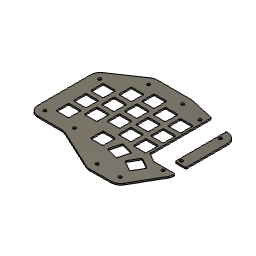
Fifi_Case_v6 (Autodesk Fusion 360 design; units mm, degrees)
Autodesk Fusion 360 part; units mm, degrees
(part 1 of 3)
sketch "top_plate" plane through (0, 0, 0) normal (0, 1, 0) x (1, 0, 0)
  arc A0 (-12.05, -31.06) -> (-13.05, -32.06) centre (-13.05, -31.06) cw
  arc A1 (-45.1, -12) -> (-44.1, -11) centre (-44.1, -12) cw
  arc A2 (-45.1, -4.95) -> (-44.1, -5.95) centre (-44.1, -4.95) ccw
  arc A3 (48.9038, -42.3878) -> (47.5378, -42.7538) centre (48.4038, -43.2538) ccw
  arc A4 (32.1, -35.05) -> (31.1, -34.05) centre (32.1, -34.05) cw
  line L0 (20.8727, -52.5986) -> (32.4638, -55.7044)
  arc A5 (41.5378, -53.1462) -> (41.9038, -54.5122) centre (42.4038, -53.6462) ccw
  line L1 (-25.05, 1) -> (-13.05, 1)
  line L2 (-32.1, 8.05) -> (-44.1, 8.05)
  line L3 (-25.05, 20.05) -> (-13.05, 20.05)
  arc A6 (-25.05, -32.06) -> (-26.05, -31.06) centre (-25.05, -31.06) cw
  arc A7 (36.7944, -43.4062) -> (36.0873, -42.1814) centre (35.8285, -43.1474) ccw
  line L4 (-45.1, -24) -> (-45.1, -12)
  arc A8 (44.1, -2) -> (45.1, -3) centre (44.1, -3) cw
  arc A9 (-12.05, -12) -> (-13.05, -13) centre (-13.05, -12) cw
  arc A10 (31.1, -22.05) -> (32.1, -21.05) centre (32.1, -22.05) cw
  arc A11 (44.1, -21.05) -> (45.1, -22.05) centre (44.1, -22.05) cw
  line L5 (-32.1, -44.05) -> (-44.1, -44.05)
  arc A12 (-32.1, -30.05) -> (-31.1, -31.05) centre (-32.1, -31.05) cw
  line L6 (-44.1, -5.95) -> (-32.1, -5.95)
  line L7 (47.5378, -42.7538) -> (41.5378, -53.1462)
  line L8 (-45.1, 7.05) -> (-45.1, -4.95)
  arc A13 (-45.1, -31.05) -> (-44.1, -30.05) centre (-44.1, -31.05) cw
  line L9 (23.2714, -39.7827) -> (20.1656, -51.3738)
  arc A14 (-25.05, 6.05) -> (-26.05, 7.05) centre (-25.05, 7.05) cw
  arc A15 (-31.1, 7.05) -> (-32.1, 8.05) centre (-32.1, 7.05) ccw
  arc A16 (-31.1, -24) -> (-32.1, -25) centre (-32.1, -24) cw
  arc A17 (32.4638, -55.7044) -> (33.6886, -54.9973) centre (32.7226, -54.7385) ccw
  line L10 (26.1407, -56.1073) -> (17.1311, -53.6931)
  arc A18 (-26.05, 0) -> (-25.05, 1) centre (-25.05, 0) cw
  line L11 (-31.1, -12) -> (-31.1, -24)
  line L12 (44.1, 3.05) -> (32.1, 3.05)
  line L13 (33.6886, -54.9973) -> (36.7944, -43.4062)
  arc A19 (-12.05, 7.05) -> (-13.05, 6.05) centre (-13.05, 7.05) cw
  line L14 (-8.525, 28.075) -> (0, 28.075)
  line L15 (-13.05, 6.05) -> (-25.05, 6.05)
  line L16 (-45.1, -43.05) -> (-45.1, -31.05)
  line L17 (-12.05, 0) -> (-12.05, -12)
  arc A20 (45.1, 4.05) -> (44.1, 3.05) centre (44.1, 4.05) cw
  arc A21 (-13.05, -18.06) -> (-12.05, -19.06) centre (-13.05, -19.06) cw
  line L18 (-12.05, -19.06) -> (-12.05, -31.06)
  arc A22 (-13.05, 1) -> (-12.05, 0) centre (-13.05, 0) cw
  arc A23 (45.1, -15) -> (44.1, -16) centre (44.1, -15) cw
  arc A24 (-26.05, -19.06) -> (-25.05, -18.06) centre (-25.05, -19.06) cw
  line L19 (41.9038, -54.5122) -> (52.2962, -60.5122)
  line L20 (-25.05, -18.06) -> (-13.05, -18.06)
  arc A25 (-25.05, -13) -> (-26.05, -12) centre (-25.05, -12) cw
  line L21 (31.1, -34.05) -> (31.1, -22.05)
  arc A26 (-44.1, -44.05) -> (-45.1, -43.05) centre (-44.1, -43.05) cw
  line L22 (-26.05, 7.05) -> (-26.05, 19.05)
  line L23 (32.1, -2) -> (44.1, -2)
  arc A27 (-44.1, -25) -> (-45.1, -24) centre (-44.1, -24) cw
  line L24 (-13.05, -13) -> (-25.05, -13)
  line L25 (-31.1, -4.95) -> (-31.1, 7.05)
  line L26 (44.1, -16) -> (32.1, -16)
  arc A28 (31.1, -3) -> (32.1, -2) centre (32.1, -3) cw
  arc A29 (24.4962, -39.0756) -> (23.2714, -39.7827) centre (24.2374, -40.0415) ccw
  line L27 (36.0873, -42.1814) -> (24.4962, -39.0756)
  line L28 (-26.05, -12) -> (-26.05, 0)
  arc A30 (-32.1, -5.95) -> (-31.1, -4.95) centre (-32.1, -4.95) ccw
  arc A31 (-31.1, -43.05) -> (-32.1, -44.05) centre (-32.1, -43.05) cw
  arc A32 (45.1, -34.05) -> (44.1, -35.05) centre (44.1, -34.05) cw
  line L29 (-44.1, -11) -> (-32.1, -11)
  arc A33 (59.6622, -49.7538) -> (59.2962, -48.3878) centre (58.7962, -49.2538) ccw
  line L30 (-31.1, -31.05) -> (-31.1, -43.05)
  line L31 (44.1, -35.05) -> (32.1, -35.05)
  line L32 (-26.05, -31.06) -> (-26.05, -19.06)
  line L33 (0, 28.075) -> (8.525, 28.075)
  arc A34 (9.025, 22.075) -> (9.525, 21.575) centre (9.525, 22.075) ccw
  arc A35 (-28.575, -34.075) -> (-29.075, -34.575) centre (-28.575, -34.575) ccw
  line L34 (59.2962, -48.3878) -> (48.9038, -42.3878)
  line L35 (9.025, 27.575) -> (9.025, 22.075)
  arc A36 (-32.1, -11) -> (-31.1, -12) centre (-32.1, -12) cw
  line L36 (-32.1, -25) -> (-44.1, -25)
  line L37 (45.1, 16.05) -> (45.1, 4.05)
  line L38 (45.1, -22.05) -> (45.1, -34.05)
  arc A37 (-44.1, 8.05) -> (-45.1, 7.05) centre (-44.1, 7.05) ccw
  line L39 (-12.05, 19.05) -> (-12.05, 7.05)
  line L40 (32.1, -21.05) -> (44.1, -21.05)
  line L41 (45.1, -3) -> (45.1, -15)
  arc A38 (-26.05, 19.05) -> (-25.05, 20.05) centre (-25.05, 19.05) cw
  line L42 (-13.05, -32.06) -> (-25.05, -32.06)
  arc A39 (20.1656, -51.3738) -> (20.8727, -52.5986) centre (21.1315, -51.6326) ccw
  arc A40 (-13.05, 20.05) -> (-12.05, 19.05) centre (-13.05, 19.05) cw
  arc A41 (65.131, -43.3338) -> (65.314, -44.0168) centre (64.881, -43.7668) cw
  line L43 (-44.1, -30.05) -> (-32.1, -30.05)
  arc A42 (52.2962, -60.5122) -> (53.6622, -60.1462) centre (52.7962, -59.6462) ccw
  arc A43 (13.05, -13.5) -> (12.05, -12.5) centre (13.05, -12.5) cw
  arc A44 (13.05, 5.55) -> (12.05, 6.55) centre (13.05, 6.55) cw
  line L44 (-19.05, 22.075) -> (-9.525, 22.075)
  line L45 (25.05, 5.55) -> (13.05, 5.55)
  arc A45 (-7, 25.05) -> (-6, 26.05) centre (-6, 25.05) cw
  line L46 (7, 25.05) -> (7, 13.05)
  line L47 (12.05, 6.55) -> (12.05, 18.55)
  arc A46 (-29.075, -45.575) -> (-29.575, -46.075) centre (-29.575, -45.575) cw
  line L48 (26.05, 18.55) -> (26.05, 6.55)
  arc A47 (7, -6) -> (6, -7) centre (6, -6) cw
  arc A48 (25.05, -18.55) -> (26.05, -19.55) centre (25.05, -19.55) cw
  line L49 (7, -13.05) -> (7, -25.05)
  line L50 (19.05, 21.575) -> (27.575, 21.575)
  line L51 (6, 12.05) -> (-6, 12.05)
  arc A49 (6, -12.05) -> (7, -13.05) centre (6, -13.05) cw
  arc A50 (-28.075, 21.575) -> (-27.575, 22.075) centre (-27.575, 21.575) cw
  arc A51 (-6, 12.05) -> (-7, 13.05) centre (-6, 13.05) cw
  arc A52 (32.1, -16) -> (31.1, -15) centre (32.1, -15) cw
  arc A53 (35.6328, -58.7212) -> (35.1504, -58.5214) centre (34.6328, -60.4533) ccw
  arc A54 (25.05, 0.5) -> (26.05, -0.5) centre (25.05, -0.5) cw
  line L52 (-46.625, 10.075) -> (-38.1, 10.075)
  arc A55 (8.525, 28.075) -> (9.025, 27.575) centre (8.525, 27.575) cw
  arc A56 (47.125, -32.3607) -> (47.625, -33.2267) centre (48.125, -32.3607) ccw
  line L53 (13.286, -51.6) -> (1.286, -51.6)
  line L54 (14.286, -38.6) -> (14.286, -50.6)
  arc A57 (1.286, -51.6) -> (0.286, -50.6) centre (1.286, -50.6) cw
  arc A58 (12.05, -0.5) -> (13.05, 0.5) centre (13.05, -0.5) cw
  arc A59 (26.05, -31.55) -> (25.05, -32.55) centre (25.05, -31.55) cw
  line L55 (7.2859, -53.625) -> (-1.408, -53.625)
  line L56 (-28.075, 10.575) -> (-28.075, 21.575)
  arc A60 (-7, -13.05) -> (-6, -12.05) centre (-6, -13.05) cw
  line L57 (26.05, -19.55) -> (26.05, -31.55)
  line L58 (53.6622, -60.1462) -> (59.6622, -49.7538)
  line L59 (-6, 26.05) -> (6, 26.05)
  arc A61 (27.575, 21.575) -> (28.075, 21.075) centre (27.575, 21.075) cw
  arc A62 (12.05, 18.55) -> (13.05, 19.55) centre (13.05, 18.55) cw
  line L60 (-6, -12.05) -> (6, -12.05)
  line L61 (-29.575, -46.075) -> (-38.1, -46.075)
  line L62 (16.6134, -53.625) -> (7.2859, -53.625)
  arc A63 (6, 26.05) -> (7, 25.05) centre (6, 25.05) cw
  arc A64 (13.286, -37.6) -> (14.286, -38.6) centre (13.286, -38.6) cw
  arc A65 (14.286, -50.6) -> (13.286, -51.6) centre (13.286, -50.6) cw
  line L63 (47.625, -33.2267) -> (49.4993, -34.3088)
  line L64 (13.05, 19.55) -> (25.05, 19.55)
  line L65 (1.286, -37.6) -> (13.286, -37.6)
  arc A66 (46.625, 19.075) -> (47.125, 18.575) centre (46.625, 18.575) cw
  line L66 (13.05, 0.5) -> (25.05, 0.5)
  arc A67 (-46.625, -46.075) -> (-47.125, -45.575) centre (-46.625, -45.575) cw
  line L67 (7, 6) -> (7, -6)
  line L68 (49.4993, -34.3088) -> (65.131, -43.3338)
  line L69 (-29.075, -34.575) -> (-29.075, -45.575)
  line L70 (-9.025, 22.575) -> (-9.025, 27.575)
  line L71 (-47.125, -45.575) -> (-47.125, 9.575)
  arc A68 (-28.575, 10.075) -> (-28.075, 10.575) centre (-28.575, 10.575) ccw
  arc A69 (51.7765, -67.4645) -> (51.0935, -67.6475) centre (51.3435, -67.2145) cw
  arc A70 (-6, -7) -> (-7, -6) centre (-6, -6) cw
  line L72 (12.05, -31.55) -> (12.05, -19.55)
  line L73 (-38.1, -46.075) -> (-46.625, -46.075)
  line L74 (28.075, 21.075) -> (28.075, 19.575)
  arc A71 (-47.125, 9.575) -> (-46.625, 10.075) centre (-46.625, 9.575) cw
  arc A72 (28.075, 19.575) -> (28.575, 19.075) centre (28.575, 19.575) ccw
  line L75 (47.125, 18.575) -> (47.125, 18.075)
  arc A73 (-9.8958, -34.3799) -> (-10.3561, -34.075) centre (-10.3561, -34.575) ccw
  arc A74 (-6, -26.05) -> (-7, -25.05) centre (-6, -25.05) cw
  arc A75 (6, 7) -> (7, 6) centre (6, 6) cw
  line L76 (-7, -6) -> (-7, 6)
  line L77 (6, -26.05) -> (-6, -26.05)
  arc A76 (12.05, -19.55) -> (13.05, -18.55) centre (13.05, -19.55) cw
  arc A77 (7, 13.05) -> (6, 12.05) centre (6, 13.05) cw
  circle A78 centre (-2.921, -36.703) radius 1
  line L78 (25.05, -13.5) -> (13.05, -13.5)
  arc A79 (13.05, -32.55) -> (12.05, -31.55) centre (13.05, -31.55) cw
  arc A80 (32.1, 3.05) -> (31.1, 4.05) centre (32.1, 4.05) cw
  circle A81 centre (-26.67, -15.494) radius 1
  arc A82 (26.05, 6.55) -> (25.05, 5.55) centre (25.05, 6.55) cw
  circle A83 centre (28.067, 3.429) radius 1
  line L79 (-7, 13.05) -> (-7, 25.05)
  line L80 (28.575, 19.075) -> (38.1, 19.075)
  line L81 (-27.575, 22.075) -> (-19.05, 22.075)
  line L82 (-19.05, -34.075) -> (-28.575, -34.075)
  line L83 (32.1, 17.05) -> (44.1, 17.05)
  line L84 (25.05, -32.55) -> (13.05, -32.55)
  circle A84 centre (40.259, -46.736) radius 1
  line L85 (38.1, 19.075) -> (46.625, 19.075)
  arc A85 (0.286, -38.6) -> (1.286, -37.6) centre (1.286, -38.6) cw
  line L86 (47.125, 18.075) -> (47.125, -32.3607)
  line L87 (65.314, -44.0168) -> (51.7765, -67.4645)
  arc A86 (-9.025, 27.575) -> (-8.525, 28.075) centre (-8.525, 27.575) cw
  arc A87 (-9.525, 22.075) -> (-9.025, 22.575) centre (-9.525, 22.575) ccw
  line L88 (31.1, 4.05) -> (31.1, 16.05)
  line L89 (6, -7) -> (-6, -7)
  arc A88 (25.05, 19.55) -> (26.05, 18.55) centre (25.05, 18.55) cw
  line L90 (13.05, -18.55) -> (25.05, -18.55)
  circle A89 centre (-26.67, 3.556) radius 1
  line L91 (51.0935, -67.6475) -> (35.6328, -58.7212)
  arc A90 (31.1, 16.05) -> (32.1, 17.05) centre (32.1, 16.05) cw
  arc A91 (26.05, -12.5) -> (25.05, -13.5) centre (25.05, -12.5) cw
  arc A92 (44.1, 17.05) -> (45.1, 16.05) centre (44.1, 16.05) cw
  line L92 (-10.3561, -34.075) -> (-19.05, -34.075)
  line L93 (-6, 7) -> (6, 7)
  line L94 (-1.8683, -53.3201) -> (-9.8958, -34.3799)
  line L95 (26.05, -0.5) -> (26.05, -12.5)
  line L96 (-7, -25.05) -> (-7, -13.05)
  arc A93 (-1.408, -53.625) -> (-1.8683, -53.3201) centre (-1.408, -53.125) cw
  line L97 (-38.1, 10.075) -> (-28.575, 10.075)
  arc A94 (17.1311, -53.6931) -> (16.6134, -53.625) centre (16.6134, -55.625) ccw
  line L98 (31.1, -15) -> (31.1, -3)
  line L99 (0.286, -50.6) -> (0.286, -38.6)
  line L100 (12.05, -12.5) -> (12.05, -0.5)
  arc A95 (-7, 6) -> (-6, 7) centre (-6, 6) cw
  arc A96 (7, -25.05) -> (6, -26.05) centre (6, -25.05) cw
  line L101 (35.1504, -58.5214) -> (26.1407, -56.1073)
  line L102 (9.525, 21.575) -> (19.05, 21.575)
sketch "bottom_plate" plane through (0, 0, 0) normal (0, 1, 0) x (1, 0, 0)
  circle A0 centre (-2.921, -36.703) radius 1
  circle A1 centre (-26.67, -15.494) radius 1
  line L0 (-19.05, 22.075) -> (-9.525, 22.075)
  arc A2 (-29.075, -45.575) -> (-29.575, -46.075) centre (-29.575, -45.575) cw
  arc A3 (68.0431, 17.5728) -> (68.543, 17.0728) centre (68.043, 17.0728) cw
  line L1 (51.0935, -67.6475) -> (35.6328, -58.7212)
  line L2 (-38.1, 10.075) -> (-28.575, 10.075)
  arc A4 (51.7765, -67.4645) -> (51.0935, -67.6475) centre (51.3435, -67.2145) cw
  arc A5 (17.1311, -53.6931) -> (16.6134, -53.625) centre (16.6134, -55.625) ccw
  line L3 (7.2859, -53.625) -> (-1.408, -53.625)
  arc A6 (9.025, 22.075) -> (9.525, 21.575) centre (9.525, 22.075) ccw
  line L4 (-38.1, -46.075) -> (-46.625, -46.075)
  line L5 (47.6251, 17.575) -> (68.0431, 17.5728)
  line L6 (-10.3561, -34.075) -> (-19.05, -34.075)
  arc A7 (47.125, 18.075) -> (47.6251, 17.575) centre (47.625, 18.075) ccw
  line L7 (-46.625, 10.075) -> (-38.1, 10.075)
  arc A8 (46.625, 19.075) -> (47.125, 18.575) centre (46.625, 18.575) cw
  line L8 (-1.8683, -53.3201) -> (-9.8958, -34.3799)
  line L9 (38.1, 19.075) -> (46.625, 19.075)
  line L10 (0, 28.075) -> (8.525, 28.075)
  line L11 (-19.05, -34.075) -> (-28.575, -34.075)
  arc A9 (-9.525, 22.075) -> (-9.025, 22.575) centre (-9.525, 22.575) ccw
  line L12 (47.125, 18.575) -> (47.125, 18.075)
  arc A10 (27.575, 21.575) -> (28.075, 21.075) centre (27.575, 21.075) cw
  arc A11 (-47.125, 9.575) -> (-46.625, 10.075) centre (-46.625, 9.575) cw
  arc A12 (-1.408, -53.625) -> (-1.8683, -53.3201) centre (-1.408, -53.125) cw
  arc A13 (28.075, 19.575) -> (28.575, 19.075) centre (28.575, 19.575) ccw
  line L13 (28.075, 21.075) -> (28.075, 19.575)
  line L14 (28.575, 19.075) -> (38.1, 19.075)
  arc A14 (-9.025, 27.575) -> (-8.525, 28.075) centre (-8.525, 27.575) cw
  line L15 (68.543, 17.0728) -> (68.543, -36.2805)
  arc A15 (-9.8958, -34.3799) -> (-10.3561, -34.075) centre (-10.3561, -34.575) ccw
  circle A16 centre (28.067, 3.429) radius 1
  line L16 (26.1407, -56.1073) -> (17.1311, -53.6931)
  arc A17 (35.6328, -58.7212) -> (35.1504, -58.5214) centre (34.6328, -60.4533) ccw
  line L17 (35.1504, -58.5214) -> (26.1407, -56.1073)
  line L18 (58.4203, -55.9572) -> (51.7765, -67.4645)
  line L19 (-9.025, 22.575) -> (-9.025, 27.575)
  circle A18 centre (40.259, -46.736) radius 1
  arc A19 (-28.575, -34.075) -> (-29.075, -34.575) centre (-28.575, -34.575) ccw
  arc A20 (-28.075, 21.575) -> (-27.575, 22.075) centre (-27.575, 21.575) cw
  line L20 (9.025, 27.575) -> (9.025, 22.075)
  arc A21 (8.525, 28.075) -> (9.025, 27.575) centre (8.525, 27.575) cw
  line L21 (67.4712, -40.2805) -> (51.7765, -67.4645)
  arc A22 (68.543, -36.2805) -> (67.4712, -40.2805) centre (60.543, -36.2805) cw
  line L22 (19.05, 21.575) -> (27.575, 21.575)
  line L23 (-8.525, 28.075) -> (0, 28.075)
  arc A23 (-28.575, 10.075) -> (-28.075, 10.575) centre (-28.575, 10.575) ccw
  arc A24 (-46.625, -46.075) -> (-47.125, -45.575) centre (-46.625, -45.575) cw
  line L24 (-27.575, 22.075) -> (-19.05, 22.075)
  line L25 (-28.075, 10.575) -> (-28.075, 21.575)
  line L26 (-29.075, -34.575) -> (-29.075, -45.575)
  line L27 (-47.125, -45.575) -> (-47.125, 9.575)
  line L28 (9.525, 21.575) -> (19.05, 21.575)
  line L29 (-29.575, -46.075) -> (-38.1, -46.075)
  circle A25 centre (-26.67, 3.556) radius 1
  line L30 (16.6134, -53.625) -> (7.2859, -53.625)
sketch "key_positions" plane through (0, 0, 0) normal (0, 1, 0) x (1, 0, 0)
  line L0 (12.05, -18.55) -> (26.05, -18.55)
  line L1 (-7, -26.05) -> (7, -12.05)
  line L2 (53.1666, -61.0068) -> (41.0422, -54.0068)
  line L3 (14.2859, -37.6) -> (14.2859, -51.6)
  line L4 (31.1, -16) -> (31.1, -2)
  line L5 (-31.1, -5.95) -> (-45.1, -5.95)
  line L6 (19.9034, -52.3396) -> (23.5268, -38.8166)
  line L7 (33.4263, -55.963) -> (19.9034, -52.3396)
  line L8 (-45.1, -25) -> (-45.1, -11)
  line L9 (-31.1, -25) -> (-45.1, -25)
  line L10 (31.1, 3.05) -> (45.1, 17.05)
  line L11 (26.05, -18.55) -> (26.05, -32.55)
  line L12 (-26.05, -32.05) -> (-12.05, -18.05)
  line L13 (-45.1, -5.95) -> (-31.1, 8.05)
  line L14 (41.0422, -54.0068) -> (48.0422, -41.8825)
  line L15 (48.0422, -41.8825) -> (60.1666, -48.8825)
  line L16 (7, 26.05) -> (7, 12.05)
  line L17 (-26.05, 6.05) -> (-26.05, 20.05)
  line L18 (45.1, -2) -> (45.1, -16)
  line L19 (35.2118, -59.0555) -> (21.7414, -35.7241)
  line L20 (-12.05, -13) -> (-26.05, -13)
  line L21 (12.05, -13.5) -> (12.05, 0.5)
  line L22 (7, 12.05) -> (-7, 12.05)
  line L23 (45.1, -35.05) -> (31.1, -35.05)
  line L24 (31.1, -21.05) -> (45.1, -21.05)
  line L25 (-45.1, -11) -> (-31.1, -11)
  line L26 (-12.05, 20.05) -> (-12.05, 6.05)
  line L27 (-26.05, 6.05) -> (-12.05, 20.05)
  line L28 (-7, -26.05) -> (-7, -12.05)
  line L29 (26.05, -32.55) -> (12.05, -18.55)
  line L30 (12.05, -32.55) -> (12.05, -18.55)
  line L31 (31.1, -16) -> (45.1, -2)
  line L32 (45.1, 17.05) -> (45.1, 3.05)
  line L33 (14.2859, -51.6) -> (0.2859, -51.6)
  line L34 (-31.1, -5.95) -> (-45.1, 8.05)
  line L35 (-31.1, 8.05) -> (-31.1, -5.95)
  line L36 (31.1, 17.05) -> (45.1, 17.05)
  line L37 (-7, -7) -> (7, 7)
  line L38 (26.05, 19.55) -> (26.05, 5.55)
  line L39 (-7, 26.05) -> (7, 26.05)
  line L40 (-7, -12.05) -> (7, -12.05)
  line L41 (-45.1, -44.05) -> (-31.1, -30.05)
  line L42 (-12.05, -32.05) -> (-26.05, -32.05)
  line L43 (0.2859, -51.6) -> (14.2859, -37.6)
  line L44 (-12.05, 6.05) -> (-26.05, 20.05)
  line L45 (-26.05, -13) -> (-26.05, 1)
  line L46 (-26.05, 1) -> (-12.05, 1)
  line L47 (-26.05, -32.05) -> (-26.05, -18.05)
  line L48 (31.1, -2) -> (45.1, -2)
  line L49 (-12.05, 1) -> (-12.05, -13)
  line L50 (12.05, 19.55) -> (26.05, 19.55)
  line L51 (-31.1, -11) -> (-31.1, -25)
  line L52 (7, -26.05) -> (-7, -12.05)
  line L53 (26.05, -32.55) -> (12.05, -32.55)
  line L54 (45.1, -16) -> (31.1, -2)
  line L55 (-31.1, -30.05) -> (-31.1, -44.05)
  line L56 (7, 7) -> (7, -7)
  line L57 (7, -7) -> (-7, 7)
  line L58 (31.1, 3.05) -> (31.1, 17.05)
  line L59 (-7, 12.05) -> (7, 26.05)
  line L60 (7, -26.05) -> (-7, -26.05)
  line L61 (-26.05, 20.05) -> (-12.05, 20.05)
  line L62 (45.1, 3.05) -> (31.1, 3.05)
  line L63 (-45.1, 8.05) -> (-31.1, 8.05)
  line L64 (-31.1, -44.05) -> (-45.1, -30.05)
  line L65 (-45.1, -5.95) -> (-45.1, 8.05)
  line L66 (12.05, 5.55) -> (26.05, 19.55)
  line L67 (-7, 12.05) -> (-7, 26.05)
  line L68 (31.1, -35.05) -> (45.1, -21.05)
  line L69 (45.1, -35.05) -> (31.1, -21.05)
  line L70 (26.05, -13.5) -> (12.05, -13.5)
  line L71 (0.2859, -51.6) -> (0.2859, -37.6)
  line L72 (14.2859, -51.6) -> (0.2859, -37.6)
  line L73 (0.2859, -37.6) -> (14.2859, -37.6)
  line L74 (7, 12.05) -> (-7, 26.05)
  line L75 (-26.05, -18.05) -> (-12.05, -18.05)
  line L76 (45.1, -16) -> (31.1, -16)
  line L77 (45.1, 3.05) -> (31.1, 17.05)
  line L78 (12.05, -32.55) -> (26.05, -18.55)
  line L79 (45.1, -21.05) -> (45.1, -35.05)
  line L80 (23.5268, -38.8166) -> (37.0498, -42.4401)
  line L81 (37.0498, -42.4401) -> (33.4263, -55.963)
  line L82 (7, -12.05) -> (7, -26.05)
  line L83 (12.05, 0.5) -> (26.05, 0.5)
  line L84 (26.05, 5.55) -> (12.05, 19.55)
  line L85 (-31.1, -25) -> (-45.1, -11)
  line L86 (26.05, 0.5) -> (26.05, -13.5)
  line L87 (-7, -7) -> (-7, 7)
  line L88 (-26.05, -13) -> (-12.05, 1)
  line L89 (16.8109, -54.125) -> (-2.2391, -35.075)
  line L90 (16.8109, -54.125) -> (40.1423, -40.6546)
  line L91 (-12.05, 6.05) -> (-26.05, 6.05)
  line L92 (-45.1, -30.05) -> (-31.1, -30.05)
  line L93 (12.05, 5.55) -> (12.05, 19.55)
  line L94 (26.05, -13.5) -> (12.05, 0.5)
  line L95 (-45.1, -44.05) -> (-45.1, -30.05)
  line L96 (16.8109, -35.075) -> (-2.2391, -54.125)
  line L97 (-7, 7) -> (7, 7)
  line L98 (-31.1, -44.05) -> (-45.1, -44.05)
  line L99 (-45.1, -25) -> (-31.1, -11)
  line L100 (31.1, -35.05) -> (31.1, -21.05)
  line L101 (-12.05, -13) -> (-26.05, 1)
  line L102 (-12.05, -18.05) -> (-12.05, -32.05)
  line L103 (-12.05, -32.05) -> (-26.05, -18.05)
  line L104 (26.05, 5.55) -> (12.05, 5.55)
  line L105 (12.05, -13.5) -> (26.05, 0.5)
  line L106 (51.7096, -68.5805) -> (49.4993, -34.3088)
  line L107 (7, -7) -> (-7, -7)
  line L108 (35.2118, -59.0555) -> (65.9971, -43.8338)
  line L109 (60.1666, -48.8825) -> (53.1666, -61.0068)
  line L110 (-47.625, -27.525) -> (-28.575, -8.475)
  line L111 (49.4993, -34.3088) -> (35.2118, -59.0555)
  line L112 (28.575, 3.025) -> (9.525, 3.025)
  line L113 (-9.525, 9.525) -> (9.525, 9.525)
  line L114 (9.525, -35.075) -> (28.575, -35.075)
  line L115 (16.8109, -54.125) -> (-2.2391, -54.125)
  line L116 (51.7096, -68.5805) -> (65.9971, -43.8338)
  line L117 (35.2118, -59.0555) -> (51.7096, -68.5805)
  line L118 (35.2118, -59.0555) -> (51.7096, -68.5805)
  line L119 (21.7414, -35.7241) -> (16.8109, -54.125)
  line L120 (9.525, -9.525) -> (-9.525, -28.575)
  line L121 (28.575, 0.525) -> (47.625, 0.525)
  line L122 (-9.525, 9.525) -> (9.525, 9.525)
  line L123 (47.625, -18.525) -> (28.575, -18.525)
  line L124 (47.625, 0.525) -> (28.575, 0.525)
  line L125 (16.8109, -54.125) -> (35.2118, -59.0555)
  line L126 (-2.2391, -35.075) -> (16.8109, -35.075)
  line L127 (47.625, -18.525) -> (28.575, -18.525)
  line L128 (-47.625, -27.525) -> (-28.575, -27.525)
  line L129 (65.9971, -43.8338) -> (49.4993, -34.3088)
  line L130 (35.2118, -59.0555) -> (54.2618, -59.0555)
  line L131 (28.575, -37.575) -> (47.625, -37.575)
  line L132 (-28.575, 3.525) -> (-9.525, 3.525)
  line L133 (9.525, -28.575) -> (-9.525, -28.575)
  line L134 (-47.625, -8.475) -> (-28.575, -8.475)
  line L135 (9.525, 22.075) -> (28.575, 22.075)
  line L136 (40.1423, -40.6546) -> (21.7414, -35.7241)
  line L137 (28.575, 3.025) -> (9.525, 22.075)
  line L138 (9.525, 3.025) -> (28.575, 3.025)
  line L139 (28.575, -16.025) -> (9.525, -16.025)
  line L140 (-2.2391, -54.125) -> (-2.2391, -35.075)
  line L141 (16.8109, -54.125) -> (35.8609, -54.125)
  line L142 (9.525, 28.575) -> (-9.525, 28.575)
  line L143 (-9.525, -9.525) -> (9.525, -9.525)
  line L144 (9.525, -9.525) -> (-9.525, 9.525)
  line L145 (9.525, 9.525) -> (9.525, -9.525)
  line L146 (28.575, 3.025) -> (28.575, -16.025)
  line L147 (16.8109, -35.075) -> (16.8109, -54.125)
  line L148 (47.625, 0.525) -> (47.625, -18.525)
  line L149 (-9.525, 3.525) -> (-28.575, 22.575)
  line L150 (28.575, -35.075) -> (28.575, -16.025)
  line L151 (-28.575, -27.525) -> (-28.575, -8.475)
  line L152 (47.625, -37.575) -> (47.625, -18.525)
  line L153 (28.575, 22.075) -> (28.575, 3.025)
  line L154 (9.525, 3.025) -> (9.525, 22.075)
  line L155 (9.525, 9.525) -> (9.525, 28.575)
  line L156 (9.525, 3.025) -> (28.575, 22.075)
  line L157 (-28.575, 3.525) -> (-9.525, 22.575)
  line L158 (-28.575, -15.525) -> (-9.525, 3.525)
  line L159 (-28.575, -8.475) -> (-47.625, 10.575)
  line L160 (28.575, -18.525) -> (28.575, 0.525)
  line L161 (-28.575, 10.575) -> (-47.625, 10.575)
  line L162 (-28.575, -15.525) -> (-9.525, -15.525)
  line L163 (28.575, -16.025) -> (9.525, -16.025)
  line L164 (-28.575, -27.525) -> (-47.625, -8.475)
  line L165 (-28.575, -8.475) -> (-47.625, -8.475)
  line L166 (-9.525, -15.525) -> (-28.575, 3.525)
  line L167 (-28.575, -27.525) -> (-47.625, -46.575)
  line L168 (-47.625, -27.525) -> (-28.575, -27.525)
  line L169 (-9.525, -15.525) -> (-28.575, -15.525)
  line L170 (-28.575, 3.525) -> (-9.525, 3.525)
  line L171 (-9.525, 22.575) -> (-28.575, 22.575)
  line L172 (28.575, 19.575) -> (47.625, 19.575)
  line L173 (-9.525, -34.575) -> (-28.575, -34.575)
  line L174 (-28.575, -46.575) -> (-47.625, -46.575)
  line L175 (-9.525, -15.525) -> (-28.575, -34.575)
  line L176 (-9.525, -34.575) -> (-28.575, -15.525)
  line L177 (-9.525, -9.525) -> (9.525, -28.575)
  line L178 (9.525, -9.525) -> (-9.525, -9.525)
  line L179 (47.625, 19.575) -> (47.625, 0.525)
  line L180 (-28.575, -34.575) -> (-28.575, -15.525)
  line L181 (-28.575, -46.575) -> (-47.625, -27.525)
  line L182 (-47.625, -8.475) -> (-28.575, 10.575)
  line L183 (-9.525, -9.525) -> (-9.525, 9.525)
  line L184 (9.525, -16.025) -> (9.525, -35.075)
  line L185 (9.525, 9.525) -> (-9.525, 28.575)
  line L186 (-9.525, 9.525) -> (9.525, 28.575)
  line L187 (35.2118, -59.0555) -> (40.1423, -40.6546)
  line L188 (28.575, 3.025) -> (9.525, -16.025)
  line L189 (28.575, -16.025) -> (9.525, -35.075)
  line L190 (9.525, -16.025) -> (9.525, 3.025)
  line L191 (28.575, 0.525) -> (47.625, 19.575)
  line L192 (47.625, -18.525) -> (28.575, 0.525)
  line L193 (-9.525, -15.525) -> (-9.525, -34.575)
  line L194 (-47.625, -8.475) -> (-47.625, -27.525)
  line L195 (47.625, 0.525) -> (28.575, 19.575)
  line L196 (28.575, 0.525) -> (28.575, 19.575)
  line L197 (47.625, -37.575) -> (28.575, -18.525)
  line L198 (28.575, -35.075) -> (9.525, -16.025)
  line L199 (9.525, -9.525) -> (9.525, -28.575)
  line L200 (-28.575, -15.525) -> (-28.575, 3.525)
  line L201 (-28.575, -27.525) -> (-28.575, -46.575)
  line L202 (-47.625, -46.575) -> (-47.625, -27.525)
  line L203 (-9.525, 28.575) -> (-9.525, 9.525)
  line L204 (-9.525, 3.525) -> (-9.525, 22.575)
  line L205 (-28.575, 22.575) -> (-28.575, 3.525)
  line L206 (-9.525, -9.525) -> (9.525, 9.525)
  line L207 (28.575, -18.525) -> (47.625, 0.525)
  line L208 (-9.525, -28.575) -> (-9.525, -9.525)
  line L209 (-47.625, 10.575) -> (-47.625, -8.475)
  line L210 (-9.525, 3.525) -> (-9.525, -15.525)
  line L211 (-28.575, -8.475) -> (-28.575, 10.575)
  line L212 (47.625, -18.525) -> (28.575, -37.575)
  line L213 (28.575, -16.025) -> (9.525, 3.025)
  line L214 (28.575, -18.525) -> (28.575, -37.575)
sketch "hard_base" plane through (0, 0, 0) normal (0, 1, 0) x (1, 0, 0)
  line L0 (-55.125, 14.4904) -> (-20.8612, 36.075)
  line L1 (-20.8612, 36.075) -> (9.7152, 36.075)
  line L2 (9.7152, 36.075) -> (76.543, 24.285)
  line L3 (76.543, 24.285) -> (76.543, -36.5677)
  line L4 (76.543, -36.5677) -> (54.9316, -73.9998)
  line L5 (54.9316, -73.9998) -> (31.9391, -73.9998)
  line L6 (-55.125, -49.4213) -> (-55.125, 14.4904)
  line L7 (31.9391, -73.9998) -> (-55.125, -49.4213)
sketch "OLEDstandin" plane through (0, 0, 0) normal (0, 1, 0) x (1, 0, 0)
  line L0 (68.543, 17.0728) -> (50.6044, 17.0728)
  line L1 (50.6044, 17.0728) -> (50.6044, -29.8845)
  line L2 (50.6044, -29.8845) -> (68.543, -29.8845)
  line L3 (68.543, -29.8845) -> (68.543, 17.0728)
  point P0 (68.543, 17.0728)
  constraint horizontal L0
  constraint horizontal L2
  constraint coincident P0 L0.start
sketch "plate_outline" plane through (0, 0, 0) normal (0, 1, 0) x (1, 0, 0)
  line L0 (-18.6222, 41.0765) -> (18.4843, 41.0734)
  line L1 (79.7028, -45.0985) -> (61.8222, -76.0618)
  line L2 (53.2987, -81.06) -> (29.1948, -81.3885)
  line L3 (-60.125, -49.075) -> (-60.125, 9.652)
  line L4 (-47.625, -8.475) -> (-47.625, -27.525)
  line L5 (-17.8516, 28.5764) -> (16.2008, 28.5736) construction
  line L6 (68.543, -29.8845) -> (68.543, 17.0728) construction
  line L7 (49.4503, -72.4899) -> (68.7483, -39.0722) construction
  line L8 (-50.125, -59.075) -> (-23.4871, -59.075)
  line L9 (-28.575, -46.575) -> (-47.625, -46.575) construction
  line L10 (-2.2391, -54.125) -> (-2.2391, -35.075) construction
  line L11 (24.8527, -80.462) -> (-19.2813, -60.0025)
  line L12 (-55.7487, 17.9209) -> (-24.2468, 39.3454)
  arc A0 (-55.7487, 17.9209) -> (-60.125, 9.652) centre (-50.125, 9.652) ccw
  arc A1 (-18.6222, 41.0765) -> (-24.2468, 39.3454) centre (-18.6231, 31.0765) ccw
  arc A2 (20.6567, 40.8344) -> (18.4843, 41.0734) centre (18.4835, 31.0734) ccw
  arc A3 (81.043, 19.3715) -> (73.2162, 29.1325) centre (71.043, 19.3715) ccw
  arc A4 (79.7028, -45.0985) -> (81.043, -40.0977) centre (71.043, -40.0977) ccw
  arc A5 (53.2987, -81.06) -> (61.8222, -76.0618) centre (53.1625, -71.0609) ccw
  arc A6 (24.8527, -80.462) -> (29.1948, -81.3885) centre (29.0585, -71.3894) ccw
  arc A7 (-19.2813, -60.0025) -> (-23.4871, -59.075) centre (-23.4871, -69.075) ccw
  arc A8 (-60.125, -49.075) -> (-50.125, -59.075) centre (-50.125, -49.075) ccw
  line L13 (47.625, 34.0283) -> (47.625, -32.5721)
  line L14 (57.6205, -38.7668) -> (80.043, -38.7668)
  line L15 (20.6567, 40.8344) -> (46.8423, 35.0044)
  line L16 (70.2867, 29.7847) -> (73.2162, 29.1325)
  line L17 (81.043, 19.3715) -> (81.043, -25.8559)
  line L18 (81.043, -39.7668) -> (81.043, -40.0977)
  line L19 (69.2205, -25.8646) -> (69.0694, 28.8059)
  line L20 (70.2211, -26.8618) -> (80.0436, -26.8559)
  line L21 (48.1249, -33.4381) -> (57.1204, -38.6328)
  line L22 (68.7213, -39.119) -> (68.7205, -38.7668)
  arc A9 (47.625, 34.0283) -> (46.8423, 35.0044) centre (46.625, 34.0283) ccw
  arc A10 (47.625, -32.5721) -> (48.1249, -33.4381) centre (48.625, -32.5721) ccw
  arc A11 (57.1204, -38.6328) -> (57.6205, -38.7668) centre (57.6205, -37.7668) ccw
  arc A12 (81.043, -39.7668) -> (80.043, -38.7668) centre (80.043, -39.7668) ccw
  arc A13 (80.0436, -26.8559) -> (81.043, -25.8559) centre (80.043, -25.8559) ccw
  arc A14 (69.2205, -25.8646) -> (70.2211, -26.8618) centre (70.2205, -25.8618) ccw
  arc A15 (70.2867, 29.7847) -> (69.0694, 28.8059) centre (70.0694, 28.8086) ccw
  circle A16 centre (72.2122, -22.8606) radius 1.7
  circle A17 centre (72.2122, -22.8606) radius 1.1
  circle A18 centre (72.0934, 20.1391) radius 1.7
  circle A19 centre (72.0934, 20.1391) radius 1.1
  circle A20 centre (71.1231, -41.9588) radius 1.1
  circle A21 centre (71.1231, -41.9588) radius 1.7
  circle A22 centre (53.7342, -72.0705) radius 1.7
  circle A23 centre (53.7342, -72.0705) radius 1.1
  circle A24 centre (28.4977, -72.2317) radius 1.7
  circle A25 centre (28.4977, -72.2317) radius 1.1
  circle A26 centre (-18.212, -50.5781) radius 1.7
  circle A27 centre (-18.212, -50.5781) radius 1.1
  circle A28 centre (-51.125, -50.075) radius 1.7
  circle A29 centre (-51.125, -50.075) radius 1.1
  circle A30 centre (-51.125, 10.1813) radius 1.7
  circle A31 centre (-51.125, 10.1813) radius 1.1
  circle A32 centre (-18.9309, 32.0765) radius 1.7
  circle A33 centre (-18.9309, 32.0765) radius 1.1
  circle A34 centre (18.5935, 32.0734) radius 1.7
  circle A35 centre (18.5935, 32.0734) radius 1.1
  circle A36 centre (43.1794, 26.5995) radius 1.7
  circle A37 centre (43.1794, 26.5995) radius 1.1
  arc A38 (80.543, 19.3715) -> (73.1075, 28.6444) centre (71.043, 19.3715) ccw
  line L23 (80.543, 19.3715) -> (80.543, -25.8607)
  arc A39 (79.293, 19.3715) -> (72.8359, 27.4243) centre (71.043, 19.3715) ccw
  line L24 (79.293, 19.3715) -> (79.293, -25.8607)
  arc A40 (75.543, 19.3715) -> (72.0209, 23.7639) centre (71.043, 19.3715) ccw
  line L25 (75.543, 19.3715) -> (75.543, -25.8607)
  arc A41 (79.543, -26.8607) -> (80.543, -25.8607) centre (79.543, -25.8607) ccw
  arc A42 (78.293, -26.8607) -> (79.293, -25.8607) centre (78.293, -25.8607) ccw
  arc A43 (74.543, -26.8607) -> (75.543, -25.8607) centre (74.543, -25.8607) ccw
  line L26 (70.2867, 29.7847) -> (70.2867, 22.8349) construction
  arc A44 (70.7856, 29.3963) -> (69.5691, 28.4178) centre (70.5691, 28.42) ccw
  arc A45 (70.785, 28.1464) -> (69.5691, 27.1678) centre (70.5691, 27.17) ccw
  line L27 (72.8359, 27.4243) -> (70.785, 28.1464)
  arc A46 (70.2803, 24.3774) -> (69.5691, 23.4178) centre (70.5691, 23.42) ccw
  line L28 (72.0209, 23.7639) -> (70.2803, 24.3774)
  line L29 (73.1075, 28.6444) -> (70.7856, 29.3963)
  line L30 (20.548, 40.3463) -> (46.7337, 34.5163)
  arc A47 (20.548, 40.3463) -> (18.4843, 40.5734) centre (18.4835, 31.0734) ccw
  line L31 (-18.6223, 40.5765) -> (18.4843, 40.5734)
  arc A48 (-18.6223, 40.5765) -> (-23.9656, 38.9319) centre (-18.6231, 31.0765) ccw
  line L32 (-55.4675, 17.5074) -> (-23.9656, 38.9319)
  arc A49 (-55.4675, 17.5074) -> (-59.625, 9.652) centre (-50.125, 9.652) ccw
  line L33 (-59.625, -49.075) -> (-59.625, 9.652)
  arc A50 (-59.625, -49.075) -> (-50.125, -58.575) centre (-50.125, -49.075) ccw
  line L34 (-50.125, -58.575) -> (-23.4871, -58.575)
  arc A51 (-19.071, -59.5488) -> (-23.4871, -58.575) centre (-23.4871, -69.075) ccw
  line L35 (25.063, -80.0083) -> (-19.071, -59.5488)
  arc A52 (25.063, -80.0083) -> (29.1879, -80.8885) centre (29.0585, -71.3894) ccw
  line L36 (53.2919, -80.5601) -> (29.1879, -80.8885)
  arc A53 (53.2919, -80.5601) -> (61.3893, -75.8117) centre (53.1625, -71.0609) ccw
  line L37 (79.2698, -44.8485) -> (61.3893, -75.8117)
  arc A54 (79.2698, -44.8485) -> (80.543, -40.0977) centre (71.043, -40.0977) ccw
  arc A55 (78.1873, -44.2234) -> (79.293, -40.0977) centre (71.043, -40.0977) ccw
  line L38 (78.1873, -44.2234) -> (60.3068, -75.1866)
  arc A56 (53.2749, -79.3102) -> (60.3068, -75.1866) centre (53.1625, -71.0609) ccw
  line L39 (53.2749, -79.3102) -> (29.1709, -79.6387)
  arc A57 (25.5887, -78.8743) -> (29.1709, -79.6387) centre (29.0585, -71.3894) ccw
  line L40 (25.5887, -78.8743) -> (-18.5453, -58.4148)
  arc A58 (-18.5453, -58.4148) -> (-23.4871, -57.325) centre (-23.4871, -69.075) ccw
  line L41 (-50.125, -57.325) -> (-23.4871, -57.325)
  arc A59 (-58.375, -49.075) -> (-50.125, -57.325) centre (-50.125, -49.075) ccw
  line L42 (-58.375, -49.075) -> (-58.375, 9.652)
  arc A60 (-54.7645, 16.4738) -> (-58.375, 9.652) centre (-50.125, 9.652) ccw
  line L43 (-54.7645, 16.4738) -> (-23.2626, 37.8983)
  arc A61 (-18.6224, 39.3265) -> (-23.2626, 37.8983) centre (-18.6231, 31.0765) ccw
  line L44 (-18.6224, 39.3265) -> (18.4842, 39.3234)
  arc A62 (20.2764, 39.1262) -> (18.4842, 39.3234) centre (18.4835, 31.0734) ccw
  line L45 (20.2764, 39.1262) -> (46.462, 33.2962)
  arc A63 (74.9399, -42.3481) -> (75.543, -40.0977) centre (71.043, -40.0977) ccw
  line L46 (74.9399, -42.3481) -> (57.0594, -73.3113)
  arc A64 (53.2238, -75.5605) -> (57.0594, -73.3113) centre (53.1625, -71.0609) ccw
  line L47 (53.2238, -75.5605) -> (29.1198, -75.889)
  arc A65 (27.1659, -75.4721) -> (29.1198, -75.889) centre (29.0585, -71.3894) ccw
  line L48 (27.1659, -75.4721) -> (-16.9681, -55.0126)
  arc A66 (-16.9681, -55.0126) -> (-23.4871, -53.575) centre (-23.4871, -69.075) ccw
  line L49 (-50.125, -53.575) -> (-23.4871, -53.575)
  arc A67 (-54.625, -49.075) -> (-50.125, -53.575) centre (-50.125, -49.075) ccw
  line L50 (-54.625, -49.075) -> (-54.625, 9.652)
  arc A68 (-52.6557, 13.373) -> (-54.625, 9.652) centre (-50.125, 9.652) ccw
  line L51 (-52.6557, 13.373) -> (-21.1537, 34.7975)
  arc A69 (-18.6227, 35.5765) -> (-21.1537, 34.7975) centre (-18.6231, 31.0765) ccw
  line L52 (-18.6227, 35.5765) -> (18.4839, 35.5734)
  arc A70 (19.4614, 35.4658) -> (18.4839, 35.5734) centre (18.4835, 31.0734) ccw
  line L53 (19.4614, 35.4658) -> (45.6471, 29.6358)
  line L54 (45.6471, 29.6358) -> (70.2803, 24.3774)
  line L55 (75.543, -25.8607) -> (75.543, -40.0977)
  point P0 (51.7096, -68.5805)
  point P1 (-2.2391, -54.125)
  point P2 (64.881, -43.7668)
  dimension "d42" = 12.5
  dimension "d43" = 12.5
  dimension "d44" = 12.5
  dimension "d45" = 12.5
  dimension "d46" = 12.5
  dimension "d48" = 12.5
  dimension "d53" = 12.5
  dimension "d55" = 10
  dimension "d56" = 5
  dimension "d58" = 1
  dimension "d59" = 3.4
  dimension "d60" = 3
  dimension "d61" = 4
  dimension "d62" = 2.2
  dimension "d63" = 3.4
  dimension "d64" = 2.2
  dimension "d65" = 3.4
  dimension "d66" = 2.2
  dimension "d68" = 3.4
  dimension "d69" = 2.2
  dimension "d72" = 9
  dimension "d73" = 3.4
  dimension "d74" = 2.2
  dimension "d75" = 3.4
  dimension "d76" = 2.2
  dimension "d78" = 3.4
  dimension "d79" = 2.2
  dimension "d80" = 9
  dimension "d81" = 9
  dimension "d82" = 3.4
  dimension "d83" = 2.2
  dimension "d84" = 9
  dimension "d85" = 9
  dimension "d86" = 3.4
  dimension "d87" = 2.2
  dimension "d88" = 9
  dimension "d89" = 9
  dimension "d90" = 3.4
  dimension "d91" = 2.2
  dimension "d92" = 3.4
  dimension "d93" = 2.2
  dimension "d94" = 9
  dimension "d100" = 9
  dimension "d101" = 9
  dimension "d102" = 9
  dimension "d103" = 9
  dimension "d104" = 9
  dimension "d105" = 9
  dimension "d130" = 1.75
  dimension "d131" = 5.5
  dimension "d139" = 3
  constraint parallel L0 L5
  constraint parallel L6 L17
  constraint parallel L1 L7
  constraint perpendicular L3 L8
  constraint tangent L3 A0
  constraint tangent L12 A0
  constraint tangent L12 A1
  constraint tangent L0 A1
  constraint equal A0 A1
  constraint tangent L0 A2
  constraint tangent A2 L15
  constraint equal A0 A2
  constraint tangent A3 L15
  constraint tangent A3 L17
  constraint equal A0 A3
  constraint tangent A4 L17
  constraint tangent L1 A4
  constraint equal A0 A4
  constraint tangent L1 A5
  constraint tangent L2 A5
  constraint equal A0 A5
  constraint tangent L2 A6
  constraint tangent L11 A6
  constraint equal A0 A6
  constraint tangent L11 A7
  constraint tangent L8 A7
  constraint equal A0 A7
  constraint tangent L8 A8
  constraint tangent L3 A8
  constraint equal A0 A8
  constraint parallel L6 L13
  constraint perpendicular L1 L21
  constraint perpendicular L14 L17
  constraint collinear L15 L16
  constraint collinear L17 L18
  constraint coincident L14 L22.end
  constraint coincident L7 L22.start
  constraint tangent L15 A9
  constraint tangent L13 A9
  constraint tangent L13 A10
  constraint tangent L21 A10
  constraint equal A9 A10
  constraint tangent L21 A11
  constraint tangent L14 A11
  constraint equal A9 A11
  constraint tangent L18 A12
  constraint tangent L14 A12
  constraint equal A9 A12
  constraint tangent L17 A13
  constraint tangent L20 A13
  constraint equal A9 A13
  constraint tangent L20 A14
  constraint tangent L19 A14
  constraint equal A9 A14
  constraint tangent L16 A15
  constraint tangent L19 A15
  constraint equal A9 A15
  constraint concentric A16 A17
  constraint concentric A18 A19
  constraint concentric A20 A21
  constraint concentric A22 A23
  constraint concentric A24 A25
  constraint concentric A26 A27
  constraint concentric A28 A29
  constraint concentric A30 A31
  constraint concentric A32 A33
  constraint concentric A34 A35
  constraint concentric A36 A37
  constraint vertical L26
  constraint concentric A3 A40
  constraint parallel L17 L25
  constraint tangent A40 L25
  constraint concentric A3 A39
  constraint parallel L17 L24
  constraint tangent A39 L24
  constraint concentric A3 A38
  constraint parallel L17 L23
  constraint tangent A38 L23
  constraint tangent A63 L55
  measures "d42" distance of L3 L4
  measures "d43" distance of L0 L5
  measures "d44" distance of L6 L17
  measures "d45" distance of L1 L7
  measures "d46" distance of L2 P0
  measures "d48" distance of L8 L9
  measures "d53" distance of P1 L11
  measures "d55" radius of A0
  measures "d56" distance of L14 P2
  measures "d58" radius of A9
  measures "d59" diameter of A16
  measures "d60" distance of L19 A16.centre
  measures "d61" distance of L20 A16.centre
  measures "d62" diameter of A17
  measures "d63" diameter of A18
  measures "d64" diameter of A19
  measures "d65" diameter of A21
  measures "d66" diameter of A20
  measures "d68" diameter of A22
  measures "d69" diameter of A23
  measures "d72" distance of L2.start A22.centre
  measures "d73" diameter of A24
  measures "d74" diameter of A25
  measures "d75" diameter of A26
  measures "d76" diameter of A27
  measures "d78" diameter of A28
  measures "d79" diameter of A29
  measures "d80" distance of L3 A28.centre
  measures "d81" distance of L8 A28.centre
  measures "d82" diameter of A30
  measures "d83" diameter of A31
  measures "d84" distance of L12 A30.centre
  measures "d85" distance of L3 A30.centre
  measures "d86" diameter of A32
  measures "d87" diameter of A33
  measures "d88" distance of L0 A32.centre
  measures "d89" distance of L12 A32.centre
  measures "d90" diameter of A34
  measures "d91" diameter of A35
  measures "d92" diameter of A36
  measures "d93" diameter of A37
  measures "d94" distance of L15 A36.centre
  measures "d100" vertical distance of L0.end A34.centre
  measures "d101" distance of L15 A34.centre
  measures "d102" distance of L1 A22.centre
  measures "d103" distance of L1 A20.centre
  measures "d104" distance of L11 A24.centre
  measures "d105" distance of L11 A26.centre
  measures "d139" distance of L19 A18.centre